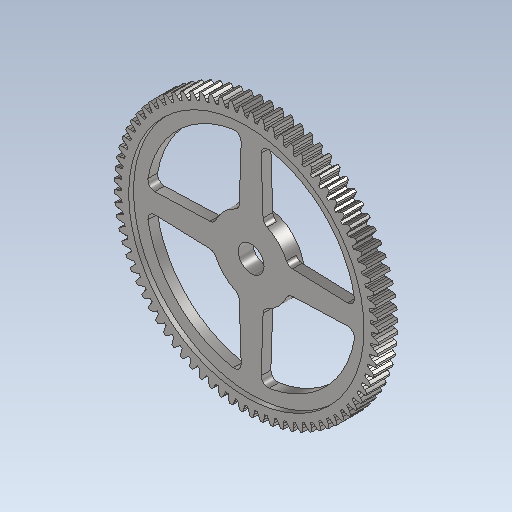
# Autodesk Inventor part: ｍ0.5歯数80焼結ギアd4
Saved by Autodesk Inventor 2020.2 (Build 242310000, 310)
## iProperties
Created: 2020-02-25
Part Number: ｍ0.5歯数80焼結ギアd4
Material: 鋼、炭素鋼
Document SubType Name: Modeling
Designer: aoyam
Density: 7.85 g/cm^3
Appearance: 半つや出し
Mass: 10.8522 g
Surface Area: 26.0429 cm^2
Volume: 1.38245 cm^3
Author: aoyam
Autodesk Inventor part; units mm, degrees
(part 1 of 4)
ref_plane "YZ Plane" through (0, 0, 0) normal (1, 0, 0) x (0, 1, 0)
ref_plane "XZ Plane" through (0, 0, 0) normal (0, 1, 0) x (-1, 0, 0)
ref_plane "XY Plane" through (0, 0, 0) normal (0, 0, 1) x (1, 0, 0)
sketch "スケッチ1" plane through (0, 0, 0) normal (0, 0, 1) x (1, 0, 0)
  arc A0 (4.5173, 26.1611) -> (4.4289, 25.8607) centre (9.5285, 24.5237) ccw
  arc A1 (4.6511, 26.5317) -> (4.5173, 26.1611) centre (10.6083, 24.1715) ccw
  arc A2 (4.8445, 26.9777) -> (4.6511, 26.5317) centre (11.7052, 23.7374) ccw
  arc A3 (4.0497, 25.8607) -> (3.9613, 26.1611) centre (-1.0499, 24.5237) ccw
  arc A4 (3.9613, 26.1611) -> (3.8275, 26.5317) centre (-2.1297, 24.1715) ccw
  arc A5 (3.8275, 26.5317) -> (3.6341, 26.9777) centre (-3.2265, 23.7374) ccw
  arc A6 (4.4289, 25.8607) -> (4.0497, 25.8607) centre (4.2393, 6.4866) ccw
  arc A7 (3.6341, 26.9777) -> (3.2349, 26.962) centre (4.2393, 6.4866) ccw
  arc A8 (2.9728, 26.1223) -> (2.9083, 25.8158) centre (8.097, 24.8831) ccw
  arc A9 (3.0771, 26.5022) -> (2.9728, 26.1223) centre (9.2011, 24.6167) ccw
  arc A10 (3.2349, 26.962) -> (3.0771, 26.5022) centre (10.3287, 24.27) ccw
  arc A11 (2.0283, 26.867) -> (1.6316, 26.8201) centre (4.2393, 6.4866) ccw
  arc A12 (2.2561, 26.4376) -> (2.0283, 26.867) centre (-4.557, 23.0985) ccw
  arc A13 (2.4185, 26.0787) -> (2.2561, 26.4376) centre (-3.4976, 23.6173) ccw
  arc A14 (2.9083, 25.8158) -> (2.5302, 25.7861) centre (4.2393, 6.4866) ccw
  arc A15 (2.5302, 25.7861) -> (2.4185, 26.0787) centre (-2.4488, 24.0531) ccw
  arc A16 (1.4361, 25.9624) -> (1.3958, 25.6518) centre (6.6418, 25.1291) ccw
  arc A17 (1.5103, 26.3493) -> (1.4361, 25.9624) centre (7.7634, 24.9501) ccw
  arc A18 (1.6316, 26.8201) -> (1.5103, 26.3493) centre (8.9146, 24.693) ccw
  arc A19 (0.436, 26.6307) -> (0.0443, 26.5528) centre (4.2393, 6.4866) ccw
  arc A20 (0.6968, 26.2205) -> (0.436, 26.6307) centre (-5.8332, 22.3571) ccw
  arc A21 (0.887, 25.8754) -> (0.6968, 26.2205) centre (-4.8178, 22.9575) ccw
  arc A22 (1.3958, 25.6518) -> (1.0212, 25.5925) centre (4.2393, 6.4866) ccw
  arc A23 (1.0212, 25.5925) -> (0.887, 25.8754) centre (-3.8064, 23.4742) ccw
  arc A24 (-0.0833, 25.6824) -> (-0.0991, 25.3697) centre (5.1717, 25.2601) ccw
  arc A25 (-0.0397, 26.074) -> (-0.0833, 25.6824) centre (6.3039, 25.1697) ccw
  arc A26 (0.0443, 26.5528) -> (-0.0397, 26.074) centre (7.4718, 25.0037) ccw
  arc A27 (-1.1327, 26.2702) -> (-1.5172, 26.1618) centre (4.2393, 6.4866) ccw
  arc A28 (-0.8405, 25.8817) -> (-1.1327, 26.2702) centre (-7.0474, 21.5179) ccw
  arc A29 (-0.6239, 25.5526) -> (-0.8405, 25.8817) centre (-6.0822, 22.1961) ccw
  arc A30 (-0.0991, 25.3697) -> (-0.4679, 25.2811) centre (4.2393, 6.4866) ccw
  arc A31 (-0.4679, 25.2811) -> (-0.6239, 25.5526) centre (-5.1144, 22.7906) ccw
  arc A32 (-1.576, 25.2841) -> (-1.5673, 24.9711) centre (3.6959, 25.2754) ccw
  arc A33 (-1.5633, 25.6779) -> (-1.576, 25.2841) centre (4.8317, 25.2741) ccw
  arc A34 (-1.5172, 26.1618) -> (-1.5633, 25.6779) centre (6.009, 25.2002) ccw
  arc A35 (-2.6684, 25.7878) -> (-3.0431, 25.6495) centre (4.2393, 6.4866) ccw
  arc A36 (-2.3466, 25.4234) -> (-2.6684, 25.7878) centre (-8.1919, 20.5861) ccw
  arc A37 (-2.1048, 25.1123) -> (-2.3466, 25.4234) centre (-7.2829, 21.3378) ccw
  arc A38 (-1.5673, 24.9711) -> (-1.928, 24.8539) centre (4.2393, 6.4866) ccw
  arc A39 (-1.928, 24.8539) -> (-2.1048, 25.1123) centre (-6.3648, 22.0065) ccw
  arc A40 (-3.033, 24.7699) -> (-2.9996, 24.4585) centre (2.2234, 25.1748) ccw
  arc A41 (-3.0512, 25.1635) -> (-3.033, 24.7699) centre (3.3558, 25.2627) ccw
  arc A42 (-3.0431, 25.6495) -> (-3.0512, 25.1635) centre (4.5353, 25.2814) ccw
  arc A43 (-4.1614, 25.1863) -> (-4.5242, 25.0191) centre (4.2393, 6.4866) ccw
  arc A44 (-3.8121, 24.8483) -> (-4.1614, 25.1863) centre (-9.2598, 19.5672) ccw
  arc A45 (-3.5466, 24.5571) -> (-3.8121, 24.8483) centre (-8.4126, 20.388) ccw
  arc A46 (-2.9996, 24.4585) -> (-3.35, 24.3134) centre (4.2393, 6.4866) ccw
  arc A47 (-3.35, 24.3134) -> (-3.5466, 24.5571) centre (-7.5498, 21.1266) ccw
  arc A48 (-4.445, 24.143) -> (-4.3874, 23.8351) centre (0.7634, 24.9591) ccw
  arc A49 (-4.4941, 24.5339) -> (-4.445, 24.143) centre (1.8854, 25.1355) ccw
  arc A50 (-4.5242, 25.0191) -> (-4.4941, 24.5339) centre (3.0597, 25.2466) ccw
  arc A51 (-5.6027, 24.4695) -> (-5.9512, 24.2743) centre (4.2393, 6.4866) ccw
  arc A52 (-5.2279, 24.16) -> (-5.6027, 24.4695) centre (-10.2445, 18.4678) ccw
  arc A53 (-4.9404, 23.8905) -> (-5.2279, 24.16) centre (-9.4643, 19.3525) ccw
  arc A54 (-4.3874, 23.8351) -> (-4.7253, 23.663) centre (4.2393, 6.4866) ccw
  arc A55 (-4.7253, 23.663) -> (-4.9404, 23.8905) centre (-8.6621, 20.1566) ccw
  arc A56 (-5.8036, 23.4072) -> (-5.7219, 23.1048) centre (-0.6753, 24.6294) ccw
  arc A57 (-5.8831, 23.793) -> (-5.8036, 23.4072) centre (0.4294, 24.8933) ccw
  arc A58 (-5.9512, 24.2743) -> (-5.8831, 23.793) centre (1.5915, 25.0963) ccw
  arc A59 (-6.9833, 23.6419) -> (-7.3154, 23.42) centre (4.2393, 6.4866) ccw
  arc A60 (-6.5853, 23.3627) -> (-6.9833, 23.6419) centre (-11.1399, 17.2945) ccw
  arc A61 (-6.2776, 23.1166) -> (-6.5853, 23.3627) centre (-10.4315, 18.2377) ccw
  arc A62 (-5.7219, 23.1048) -> (-6.0453, 22.9067) centre (4.2393, 6.4866) ccw
  arc A63 (-6.0453, 22.9067) -> (-6.2776, 23.1166) centre (-9.6948, 19.1022) ccw
  arc A64 (-7.1002, 22.567) -> (-6.9951, 22.272) centre (-2.0836, 24.1879) ccw
  arc A65 (-7.2097, 22.9455) -> (-7.1002, 22.567) centre (-1.003, 24.5376) ccw
  arc A66 (-7.3154, 23.42) -> (-7.2097, 22.9455) centre (0.1395, 24.8311) ccw
  arc A67 (-8.2947, 22.7085) -> (-8.6084, 22.4612) centre (4.2393, 6.4866) ccw
  arc A68 (-7.876, 22.4614) -> (-8.2947, 22.7085) centre (-11.9405, 16.0545) ccw
  arc A69 (-7.55, 22.2402) -> (-7.876, 22.4614) centre (-11.3083, 17.0504) ccw
  arc A70 (-6.9951, 22.272) -> (-7.3019, 22.0491) centre (4.2393, 6.4866) ccw
  arc A71 (-7.3019, 22.0491) -> (-7.55, 22.2402) centre (-10.6417, 17.97) ccw
  arc A72 (-8.3269, 21.6278) -> (-8.199, 21.3419) centre (-3.4529, 23.6372) ccw
  arc A73 (-8.4658, 21.9965) -> (-8.3269, 21.6278) centre (-2.4031, 24.0707) ccw
  arc A74 (-8.6084, 22.4612) -> (-8.4658, 21.9965) centre (-1.2871, 24.4529) ccw
  arc A75 (-9.5288, 21.6751) -> (-9.8221, 21.4039) centre (4.2393, 6.4866) ccw
  arc A76 (-9.0921, 21.4616) -> (-9.5288, 21.6751) centre (-12.6413, 14.7556) ccw
  arc A77 (-8.7497, 21.2667) -> (-9.0921, 21.4616) centre (-12.0892, 15.798) ccw
  arc A78 (-8.199, 21.3419) -> (-8.4873, 21.0956) centre (4.2393, 6.4866) ccw
  arc A79 (-8.4873, 21.0956) -> (-8.7497, 21.2667) centre (-11.4968, 16.7671) ccw
  arc A80 (-9.4761, 20.5952) -> (-9.3261, 20.3202) centre (-4.7748, 22.9808) ccw
  arc A81 (-9.6435, 20.9518) -> (-9.4761, 20.5952) centre (-3.7622, 23.4953) ccw
  arc A82 (-9.8221, 21.4039) -> (-9.6435, 20.9518) centre (-2.6797, 23.964) ccw
  arc A83 (-10.678, 20.548) -> (-10.9492, 20.2547) centre (4.2393, 6.4866) ccw
  arc A84 (-10.2259, 20.3695) -> (-10.678, 20.548) centre (-13.238, 13.4056) ccw
  arc A85 (-9.8693, 20.202) -> (-10.2259, 20.3695) centre (-12.7694, 14.4882) ccw
  arc A86 (-9.3261, 20.3202) -> (-9.5943, 20.0521) centre (4.2393, 6.4866) ccw
  arc A87 (-9.5943, 20.0521) -> (-9.8693, 20.202) centre (-12.2549, 15.5007) ccw
  arc A88 (-10.5408, 19.4756) -> (-10.3697, 19.2133) centre (-6.0411, 22.2227) ccw
  arc A89 (-10.7357, 19.818) -> (-10.5408, 19.4756) centre (-5.0721, 22.8151) ccw
  arc A90 (-10.9492, 20.2547) -> (-10.7357, 19.818) centre (-4.0296, 23.3672) ccw
  arc A91 (-11.7353, 19.3343) -> (-11.9826, 19.0206) centre (4.2393, 6.4866) ccw
  arc A92 (-11.2705, 19.1917) -> (-11.7353, 19.3343) centre (-13.727, 12.0131) ccw
  arc A93 (-10.9019, 19.0528) -> (-11.2705, 19.1917) centre (-13.3447, 13.129) ccw
  arc A94 (-10.3697, 19.2133) -> (-10.616, 18.9249) centre (4.2393, 6.4866) ccw
  arc A95 (-10.616, 18.9249) -> (-10.9019, 19.0528) centre (-12.9113, 14.1788) ccw
  arc A96 (-11.5143, 18.2759) -> (-11.3232, 18.0278) centre (-7.2441, 21.3676) ccw
  arc A97 (-11.7355, 18.602) -> (-11.5143, 18.2759) centre (-6.3245, 22.0342) ccw
  arc A98 (-11.9826, 19.0206) -> (-11.7355, 18.602) centre (-5.3286, 22.6664) ccw
  arc A99 (-12.694, 18.0413) -> (-12.916, 17.7092) centre (4.2393, 6.4866) ccw
  arc A100 (-12.2196, 17.9357) -> (-12.694, 18.0413) centre (-14.1052, 10.5864) ccw
  arc A101 (-11.8411, 17.8261) -> (-12.2196, 17.9357) centre (-13.8117, 11.7289) ccw
  arc A102 (-11.3232, 18.0278) -> (-11.5461, 17.721) centre (4.2393, 6.4866) ccw
  arc A103 (-11.5461, 17.721) -> (-11.8411, 17.8261) centre (-13.4619, 12.8095) ccw
  arc A104 (-12.3907, 17.0036) -> (-12.1807, 16.7712) centre (-8.3762, 20.4208) ccw
  arc A105 (-12.6368, 17.3113) -> (-12.3907, 17.0036) centre (-7.5118, 21.1574) ccw
  arc A106 (-12.916, 17.7092) -> (-12.6368, 17.3113) centre (-6.5685, 21.8658) ccw
  arc A107 (-13.5484, 16.6771) -> (-13.7436, 16.3286) centre (4.2393, 6.4866) ccw
  arc A108 (-13.0671, 16.609) -> (-13.5484, 16.6771) centre (-14.3703, 9.1345) ccw
  arc A109 (-12.6812, 16.5295) -> (-13.0671, 16.609) centre (-14.1674, 10.2965) ccw
  arc A110 (-12.1807, 16.7712) -> (-12.3789, 16.4479) centre (4.2393, 6.4866) ccw
  arc A111 (-12.3789, 16.4479) -> (-12.6812, 16.5295) centre (-13.9035, 11.4012) ccw
  arc A112 (-13.1646, 15.6664) -> (-12.937, 15.4512) centre (-9.4306, 19.388) ccw
  arc A113 (-13.434, 15.9538) -> (-13.1646, 15.6664) centre (-8.6266, 20.1902) ccw
  arc A114 (-13.7436, 16.3286) -> (-13.434, 15.9538) centre (-7.7419, 20.9705) ccw
  arc A115 (-14.2931, 15.2501) -> (-14.4604, 14.8874) centre (4.2393, 6.4866) ccw
  arc A116 (-13.8079, 15.22) -> (-14.2931, 15.2501) centre (-14.5207, 7.6662) ccw
  arc A117 (-13.417, 15.171) -> (-13.8079, 15.22) centre (-14.4095, 8.8406) ccw
  arc A118 (-12.937, 15.4512) -> (-13.1092, 15.1133) centre (4.2393, 6.4866) ccw
  arc A119 (-13.1092, 15.1133) -> (-13.417, 15.171) centre (-14.2331, 9.9626) ccw
  arc A120 (-13.8312, 14.2726) -> (-13.5874, 14.076) centre (-10.4007, 18.2757) ccw
  arc A121 (-14.1223, 14.538) -> (-13.8312, 14.2726) centre (-9.6621, 19.1385) ccw
  arc A122 (-14.4604, 14.8874) -> (-14.1223, 14.538) centre (-8.8413, 19.9858) ccw
  arc A123 (-14.9236, 13.7691) -> (-15.0618, 13.3943) centre (4.2393, 6.4866) ccw
  arc A124 (-14.4375, 13.7771) -> (-14.9236, 13.7691) centre (-14.5554, 6.1907) ccw
  arc A125 (-14.044, 13.7589) -> (-14.4375, 13.7771) centre (-14.5367, 7.3701) ccw
  arc A126 (-13.5874, 14.076) -> (-13.7326, 13.7256) centre (4.2393, 6.4866) ccw
  arc A127 (-13.7326, 13.7256) -> (-14.044, 13.7589) centre (-14.4489, 8.5025) ccw
  arc A128 (-14.3864, 12.8308) -> (-14.1279, 12.6539) centre (-11.2805, 17.0907) ccw
  arc A129 (-14.6974, 13.0725) -> (-14.3864, 12.8308) centre (-10.6119, 18.0089) ccw
  arc A130 (-15.0618, 13.3943) -> (-14.6974, 13.0725) centre (-9.8601, 18.9179) ccw
  arc A131 (-15.4359, 12.2431) -> (-15.5443, 11.8587) centre (4.2393, 6.4866) ccw
  arc A132 (-14.9519, 12.2893) -> (-15.4359, 12.2431) centre (-14.4743, 4.717) ccw
  arc A133 (-14.5582, 12.302) -> (-14.9519, 12.2893) centre (-14.5482, 5.8943) ccw
  arc A134 (-14.1279, 12.6539) -> (-14.2451, 12.2932) centre (4.2393, 6.4866) ccw
  arc A135 (-14.2451, 12.2932) -> (-14.5582, 12.302) centre (-14.5494, 7.0301) ccw
  arc A136 (-14.8267, 11.3499) -> (-14.5552, 11.1938) centre (-12.0647, 15.8404) ccw
  arc A137 (-15.1558, 11.5665) -> (-14.8267, 11.3499) centre (-11.4701, 16.8081) ccw
  arc A138 (-15.5443, 11.8587) -> (-15.1558, 11.5665) centre (-10.792, 17.7733) ccw
  arc A139 (-15.8269, 10.6817) -> (-15.9048, 10.2899) centre (4.2393, 6.4866) ccw
  arc A140 (-15.3481, 10.7656) -> (-15.8269, 10.6817) centre (-14.2777, 3.2542) ccw
  arc A141 (-14.9565, 10.8092) -> (-15.3481, 10.7656) centre (-14.4438, 4.422) ccw
  arc A142 (-14.5552, 11.1938) -> (-14.6437, 10.825) centre (4.2393, 6.4866) ccw
  arc A143 (-14.6437, 10.825) -> (-14.9565, 10.8092) centre (-14.5342, 5.5542) ccw
  arc A144 (-15.1495, 9.839) -> (-14.8666, 9.7047) centre (-12.7483, 14.5323) ccw
  arc A145 (-15.4946, 10.0291) -> (-15.1495, 9.839) centre (-12.2315, 15.5438) ccw
  arc A146 (-15.9048, 10.2899) -> (-15.4946, 10.0291) centre (-11.6312, 16.5592) ccw
  arc A147 (-16.0942, 9.0944) -> (-16.1411, 8.6977) centre (4.2393, 6.4866) ccw
  arc A148 (-15.6234, 9.2156) -> (-16.0942, 9.0944) centre (-13.967, 1.8113) ccw
  arc A149 (-15.2365, 9.2898) -> (-15.6234, 9.2156) centre (-14.2242, 2.9626) ccw
  arc A150 (-14.8666, 9.7047) -> (-14.9259, 9.3301) centre (4.2393, 6.4866) ccw
  arc A151 (-14.9259, 9.3301) -> (-15.2365, 9.2898) centre (-14.4031, 4.0842) ccw
  arc A152 (-15.3527, 8.3074) -> (-15.0602, 8.1957) centre (-13.3272, 13.1747) ccw
  arc A153 (-15.7117, 8.4699) -> (-15.3527, 8.3074) centre (-12.8914, 14.2235) ccw
  arc A154 (-16.1411, 8.6977) -> (-15.7117, 8.4699) centre (-12.3726, 15.2829) ccw
  arc A155 (-16.2361, 7.491) -> (-16.2518, 7.0918) centre (4.2393, 6.4866) ccw
  arc A156 (-15.7763, 7.6488) -> (-16.2361, 7.491) centre (-13.5441, 0.3973) ccw
  arc A157 (-15.3964, 7.7531) -> (-15.7763, 7.6488) centre (-13.8908, 1.5248) ccw
  arc A158 (-15.0602, 8.1957) -> (-15.0899, 7.8177) centre (4.2393, 6.4866) ccw
  arc A159 (-15.0899, 7.8177) -> (-15.3964, 7.7531) centre (-14.1572, 2.6289) ccw
  arc A160 (-15.4352, 6.7646) -> (-15.1348, 6.6762) centre (-13.7978, 11.7758) ccw
  arc A161 (-15.8058, 6.8984) -> (-15.4352, 6.7646) centre (-13.4456, 12.8556) ccw
  arc A162 (-16.2518, 7.0918) -> (-15.8058, 6.8984) centre (-13.0115, 13.9525) ccw
  arc A163 (-16.2518, 5.8814) -> (-16.2361, 5.4823) centre (4.2393, 6.4866) ccw
  arc A164 (-15.8058, 6.0748) -> (-16.2518, 5.8814) centre (-13.0115, -0.9792) ccw
  arc A165 (-15.4352, 6.2086) -> (-15.8058, 6.0748) centre (-13.4456, 0.1176) ccw
  arc A166 (-15.1348, 6.6762) -> (-15.1348, 6.297) centre (4.2393, 6.4866) ccw
  arc A167 (-15.1348, 6.297) -> (-15.4352, 6.2086) centre (-13.7978, 1.1974) ccw
  arc A168 (-15.3964, 5.2201) -> (-15.0899, 5.1556) centre (-14.1572, 10.3443) ccw
  arc A169 (-15.7763, 5.3244) -> (-15.3964, 5.2201) centre (-13.8908, 11.4485) ccw
  arc A170 (-16.2361, 5.4823) -> (-15.7763, 5.3244) centre (-13.5441, 12.576) ccw
  arc A171 (-16.1411, 4.2756) -> (-16.0942, 3.8789) centre (4.2393, 6.4866) ccw
  arc A172 (-15.7117, 4.5034) -> (-16.1411, 4.2756) centre (-12.3726, -2.3097) ccw
  arc A173 (-15.3527, 4.6658) -> (-15.7117, 4.5034) centre (-12.8914, -1.2503) ccw
  arc A174 (-15.0899, 5.1556) -> (-15.0602, 4.7775) centre (4.2393, 6.4866) ccw
  arc A175 (-15.0602, 4.7775) -> (-15.3527, 4.6658) centre (-13.3272, -0.2015) ccw
  arc A176 (-15.2365, 3.6834) -> (-14.9259, 3.6431) centre (-14.4031, 8.8891) ccw
  arc A177 (-15.6234, 3.7576) -> (-15.2365, 3.6834) centre (-14.2242, 10.0107) ccw
  arc A178 (-16.0942, 3.8789) -> (-15.6234, 3.7576) centre (-13.967, 11.1619) ccw
  arc A179 (-15.9048, 2.6834) -> (-15.8269, 2.2916) centre (4.2393, 6.4866) ccw
  arc A180 (-15.4946, 2.9442) -> (-15.9048, 2.6834) centre (-11.6312, -3.5859) ccw
  arc A181 (-15.1495, 3.1343) -> (-15.4946, 2.9442) centre (-12.2315, -2.5705) ccw
  arc A182 (-14.9259, 3.6431) -> (-14.8666, 3.2686) centre (4.2393, 6.4866) ccw
  arc A183 (-14.8666, 3.2686) -> (-15.1495, 3.1343) centre (-12.7483, -1.5591) ccw
  arc A184 (-14.9565, 2.164) -> (-14.6437, 2.1482) centre (-14.5342, 7.419) ccw
  arc A185 (-15.3481, 2.2076) -> (-14.9565, 2.164) centre (-14.4438, 8.5512) ccw
  arc A186 (-15.8269, 2.2916) -> (-15.3481, 2.2076) centre (-14.2777, 9.7191) ccw
  arc A187 (-15.5443, 1.1146) -> (-15.4359, 0.7301) centre (4.2393, 6.4866) ccw
  arc A188 (-15.1558, 1.4068) -> (-15.5443, 1.1146) centre (-10.792, -4.8001) ccw
  arc A189 (-14.8267, 1.6234) -> (-15.1558, 1.4068) centre (-11.4701, -3.8349) ccw
  arc A190 (-14.6437, 2.1482) -> (-14.5552, 1.7794) centre (4.2393, 6.4866) ccw
  arc A191 (-14.5552, 1.7794) -> (-14.8267, 1.6234) centre (-12.0647, -2.8671) ccw
  arc A192 (-14.5582, 0.6713) -> (-14.2451, 0.6801) centre (-14.5494, 5.9432) ccw
  arc A193 (-14.9519, 0.684) -> (-14.5582, 0.6713) centre (-14.5482, 7.079) ccw
  arc A194 (-15.4359, 0.7301) -> (-14.9519, 0.684) centre (-14.4743, 8.2563) ccw
  arc A195 (-15.0618, -0.4211) -> (-14.9236, -0.7958) centre (4.2393, 6.4866) ccw
  arc A196 (-14.6974, -0.0993) -> (-15.0618, -0.4211) centre (-9.8601, -5.9446) ccw
  arc A197 (-14.3864, 0.1425) -> (-14.6974, -0.0993) centre (-10.6119, -5.0356) ccw
  arc A198 (-14.2451, 0.6801) -> (-14.1279, 0.3194) centre (4.2393, 6.4866) ccw
  arc A199 (-14.1279, 0.3194) -> (-14.3864, 0.1425) centre (-11.2805, -4.1175) ccw
  arc A200 (-14.044, -0.7856) -> (-13.7326, -0.7523) centre (-14.4489, 4.4707) ccw
  arc A201 (-14.4375, -0.8038) -> (-14.044, -0.7856) centre (-14.5367, 5.6031) ccw
  arc A202 (-14.9236, -0.7958) -> (-14.4375, -0.8038) centre (-14.5554, 6.7826) ccw
  arc A203 (-14.4604, -1.9141) -> (-14.2931, -2.2769) centre (4.2393, 6.4866) ccw
  arc A204 (-14.1223, -1.5647) -> (-14.4604, -1.9141) centre (-8.8413, -7.0125) ccw
  arc A205 (-13.8312, -1.2993) -> (-14.1223, -1.5647) centre (-9.6621, -6.1653) ccw
  arc A206 (-13.7326, -0.7523) -> (-13.5874, -1.1027) centre (4.2393, 6.4866) ccw
  arc A207 (-13.5874, -1.1027) -> (-13.8312, -1.2993) centre (-10.4007, -5.3025) ccw
  arc A208 (-13.417, -2.1977) -> (-13.1092, -2.1401) centre (-14.2331, 3.0107) ccw
  arc A209 (-13.8079, -2.2467) -> (-13.417, -2.1977) centre (-14.4095, 4.1327) ccw
  arc A210 (-14.2931, -2.2769) -> (-13.8079, -2.2467) centre (-14.5207, 5.307) ccw
  arc A211 (-13.7436, -3.3554) -> (-13.5484, -3.7039) centre (4.2393, 6.4866) ccw
  arc A212 (-13.434, -2.9806) -> (-13.7436, -3.3554) centre (-7.7419, -7.9972) ccw
  arc A213 (-13.1646, -2.6931) -> (-13.434, -2.9806) centre (-8.6266, -7.217) ccw
  arc A214 (-13.1092, -2.1401) -> (-12.937, -2.478) centre (4.2393, 6.4866) ccw
  arc A215 (-12.937, -2.478) -> (-13.1646, -2.6931) centre (-9.4306, -6.4148) ccw
  arc A216 (-12.6812, -3.5562) -> (-12.3789, -3.4746) centre (-13.9035, 1.5721) ccw
  arc A217 (-13.0671, -3.6358) -> (-12.6812, -3.5562) centre (-14.1674, 2.6768) ccw
  arc A218 (-13.5484, -3.7039) -> (-13.0671, -3.6358) centre (-14.3703, 3.8388) ccw
  arc A219 (-12.916, -4.736) -> (-12.694, -5.0681) centre (4.2393, 6.4866) ccw
  arc A220 (-12.6368, -4.338) -> (-12.916, -4.736) centre (-6.5685, -8.8926) ccw
  arc A221 (-12.3907, -4.0303) -> (-12.6368, -4.338) centre (-7.5118, -8.1842) ccw
  arc A222 (-12.3789, -3.4746) -> (-12.1807, -3.798) centre (4.2393, 6.4866) ccw
  arc A223 (-12.1807, -3.798) -> (-12.3907, -4.0303) centre (-8.3762, -7.4475) ccw
  arc A224 (-11.8411, -4.8528) -> (-11.5461, -4.7478) centre (-13.4619, 0.1637) ccw
  arc A225 (-12.2196, -4.9624) -> (-11.8411, -4.8528) centre (-13.8117, 1.2443) ccw
  arc A226 (-12.694, -5.0681) -> (-12.2196, -4.9624) centre (-14.1052, 2.3868) ccw
  arc A227 (-11.9826, -6.0473) -> (-11.7353, -6.3611) centre (4.2393, 6.4866) ccw
  arc A228 (-11.7355, -5.6287) -> (-11.9826, -6.0473) centre (-5.3286, -9.6932) ccw
  arc A229 (-11.5143, -5.3027) -> (-11.7355, -5.6287) centre (-6.3245, -9.0609) ccw
  arc A230 (-11.5461, -4.7478) -> (-11.3232, -5.0546) centre (4.2393, 6.4866) ccw
  arc A231 (-11.3232, -5.0546) -> (-11.5143, -5.3027) centre (-7.2441, -8.3944) ccw
  arc A232 (-10.9019, -6.0795) -> (-10.616, -5.9516) centre (-12.9113, -1.2056) ccw
  arc A233 (-11.2705, -6.2185) -> (-10.9019, -6.0795) centre (-13.3447, -0.1558) ccw
  arc A234 (-11.7353, -6.3611) -> (-11.2705, -6.2185) centre (-13.727, 0.9602) ccw
  arc A235 (-10.9492, -7.2815) -> (-10.678, -7.5748) centre (4.2393, 6.4866) ccw
  arc A236 (-10.7357, -6.8447) -> (-10.9492, -7.2815) centre (-4.0296, -10.394) ccw
  arc A237 (-10.5408, -6.5023) -> (-10.7357, -6.8447) centre (-5.0721, -9.8418) ccw
  arc A238 (-10.616, -5.9516) -> (-10.3697, -6.24) centre (4.2393, 6.4866) ccw
  arc A239 (-10.3697, -6.24) -> (-10.5408, -6.5023) centre (-6.0411, -9.2495) ccw
  arc A240 (-9.8693, -7.2288) -> (-9.5943, -7.0788) centre (-12.2549, -2.5275) ccw
  arc A241 (-10.2259, -7.3962) -> (-9.8693, -7.2288) centre (-12.7694, -1.5149) ccw
  arc A242 (-10.678, -7.5748) -> (-10.2259, -7.3962) centre (-13.238, -0.4324) ccw
  arc A243 (-9.8221, -8.4307) -> (-9.5288, -8.7019) centre (4.2393, 6.4866) ccw
  arc A244 (-9.6435, -7.9786) -> (-9.8221, -8.4307) centre (-2.6797, -10.9907) ccw
  arc A245 (-9.4761, -7.6219) -> (-9.6435, -7.9786) centre (-3.7622, -10.5221) ccw
  arc A246 (-9.5943, -7.0788) -> (-9.3261, -7.347) centre (4.2393, 6.4866) ccw
  arc A247 (-9.3261, -7.347) -> (-9.4761, -7.6219) centre (-4.7748, -10.0076) ccw
  arc A248 (-8.7497, -8.2934) -> (-8.4873, -8.1224) centre (-11.4968, -3.7938) ccw
  arc A249 (-9.0921, -8.4883) -> (-8.7497, -8.2934) centre (-12.0892, -2.8247) ccw
  arc A250 (-9.5288, -8.7019) -> (-9.0921, -8.4883) centre (-12.6413, -1.7823) ccw
  arc A251 (-8.6084, -9.488) -> (-8.2947, -9.7353) centre (4.2393, 6.4866) ccw
  arc A252 (-8.4658, -9.0232) -> (-8.6084, -9.488) centre (-1.2871, -11.4797) ccw
  arc A253 (-8.3269, -8.6545) -> (-8.4658, -9.0232) centre (-2.4031, -11.0974) ccw
  arc A254 (-8.4873, -8.1224) -> (-8.199, -8.3687) centre (4.2393, 6.4866) ccw
  arc A255 (-8.199, -8.3687) -> (-8.3269, -8.6545) centre (-3.4529, -10.664) ccw
  arc A256 (-7.55, -9.267) -> (-7.3019, -9.0759) centre (-10.6417, -4.9968) ccw
  arc A257 (-7.876, -9.4881) -> (-7.55, -9.267) centre (-11.3083, -4.0772) ccw
  arc A258 (-8.2947, -9.7353) -> (-7.876, -9.4881) centre (-11.9405, -3.0813) ccw
  arc A259 (-7.3154, -10.4467) -> (-6.9833, -10.6687) centre (4.2393, 6.4866) ccw
  arc A260 (-7.2097, -9.9722) -> (-7.3154, -10.4467) centre (0.1395, -11.8579) ccw
  arc A261 (-7.1002, -9.5938) -> (-7.2097, -9.9722) centre (-1.003, -11.5644) ccw
  arc A262 (-7.3019, -9.0759) -> (-6.9951, -9.2988) centre (4.2393, 6.4866) ccw
  arc A263 (-6.9951, -9.2988) -> (-7.1002, -9.5938) centre (-2.0836, -11.2146) ccw
  arc A264 (-6.2776, -10.1434) -> (-6.0453, -9.9334) centre (-9.6948, -6.1289) ccw
  arc A265 (-6.5853, -10.3895) -> (-6.2776, -10.1434) centre (-10.4315, -5.2644) ccw
  arc A266 (-6.9833, -10.6687) -> (-6.5853, -10.3895) centre (-11.1399, -4.3212) ccw
  arc A267 (-5.9512, -11.3011) -> (-5.6027, -11.4963) centre (4.2393, 6.4866) ccw
  arc A268 (-5.8831, -10.8198) -> (-5.9512, -11.3011) centre (1.5915, -12.123) ccw
  arc A269 (-5.8036, -10.4339) -> (-5.8831, -10.8198) centre (0.4294, -11.92) ccw
  arc A270 (-6.0453, -9.9334) -> (-5.7219, -10.1316) centre (4.2393, 6.4866) ccw
  arc A271 (-5.7219, -10.1316) -> (-5.8036, -10.4339) centre (-0.6753, -11.6561) ccw
  arc A272 (-4.9404, -10.9173) -> (-4.7253, -10.6897) centre (-8.6621, -7.1833) ccw
  arc A273 (-5.2279, -11.1867) -> (-4.9404, -10.9173) centre (-9.4643, -6.3793) ccw
  arc A274 (-5.6027, -11.4963) -> (-5.2279, -11.1867) centre (-10.2445, -5.4945) ccw
  arc A275 (-4.5242, -12.0458) -> (-4.1614, -12.213) centre (4.2393, 6.4866) ccw
  arc A276 (-4.4941, -11.5606) -> (-4.5242, -12.0458) centre (3.0597, -12.2734) ccw
  arc A277 (-4.445, -11.1697) -> (-4.4941, -11.5606) centre (1.8854, -12.1622) ccw
  arc A278 (-4.7253, -10.6897) -> (-4.3874, -10.8619) centre (4.2393, 6.4866) ccw
  arc A279 (-4.3874, -10.8619) -> (-4.445, -11.1697) centre (0.7634, -11.9858) ccw
  arc A280 (-3.5466, -11.5839) -> (-3.35, -11.3401) centre (-7.5498, -8.1534) ccw
  arc A281 (-3.8121, -11.875) -> (-3.5466, -11.5839) centre (-8.4126, -7.4148) ccw
  arc A282 (-4.1614, -12.213) -> (-3.8121, -11.875) centre (-9.2598, -6.594) ccw
  arc A283 (-3.0431, -12.6763) -> (-2.6684, -12.8145) centre (4.2393, 6.4866) ccw
  arc A284 (-3.0512, -12.1902) -> (-3.0431, -12.6763) centre (4.5353, -12.3081) ccw
  arc A285 (-3.033, -11.7966) -> (-3.0512, -12.1902) centre (3.3558, -12.2894) ccw
  arc A286 (-3.35, -11.3401) -> (-2.9996, -11.4853) centre (4.2393, 6.4866) ccw
  arc A287 (-2.9996, -11.4853) -> (-3.033, -11.7966) centre (2.2234, -12.2016) ccw
  arc A288 (-2.1048, -12.139) -> (-1.928, -11.8806) centre (-6.3648, -9.0332) ccw
  arc A289 (-2.3466, -12.4501) -> (-2.1048, -12.139) centre (-7.2829, -8.3646) ccw
  arc A290 (-2.6684, -12.8145) -> (-2.3466, -12.4501) centre (-8.1919, -7.6128) ccw
  arc A291 (-1.5172, -13.1886) -> (-1.1327, -13.297) centre (4.2393, 6.4866) ccw
  arc A292 (-1.5633, -12.7046) -> (-1.5172, -13.1886) centre (6.009, -12.227) ccw
  arc A293 (-1.576, -12.3109) -> (-1.5633, -12.7046) centre (4.8317, -12.3009) ccw
  arc A294 (-1.928, -11.8806) -> (-1.5673, -11.9978) centre (4.2393, 6.4866) ccw
  arc A295 (-1.5673, -11.9978) -> (-1.576, -12.3109) centre (3.6959, -12.3021) ccw
  arc A296 (-0.6239, -12.5794) -> (-0.4679, -12.3079) centre (-5.1144, -9.8174) ccw
  arc A297 (-0.8405, -12.9085) -> (-0.6239, -12.5794) centre (-6.0822, -9.2228) ccw
  arc A298 (-1.1327, -13.297) -> (-0.8405, -12.9085) centre (-7.0474, -8.5447) ccw
  arc A299 (0.0443, -13.5796) -> (0.436, -13.6575) centre (4.2393, 6.4866) ccw
  arc A300 (-0.0397, -13.1007) -> (0.0443, -13.5796) centre (7.4718, -12.0304) ccw
  arc A301 (-0.0833, -12.7092) -> (-0.0397, -13.1007) centre (6.3039, -12.1965) ccw
  arc A302 (-0.4679, -12.3079) -> (-0.0991, -12.3964) centre (4.2393, 6.4866) ccw
  arc A303 (-0.0991, -12.3964) -> (-0.0833, -12.7092) centre (5.1717, -12.2869) ccw
  arc A304 (0.887, -12.9022) -> (1.0212, -12.6193) centre (-3.8064, -10.501) ccw
  arc A305 (0.6968, -13.2473) -> (0.887, -12.9022) centre (-4.8178, -9.9842) ccw
  arc A306 (0.436, -13.6575) -> (0.6968, -13.2473) centre (-5.8332, -9.3839) ccw
  arc A307 (1.6316, -13.8468) -> (2.0283, -13.8938) centre (4.2393, 6.4866) ccw
  arc A308 (1.5103, -13.3761) -> (1.6316, -13.8468) centre (8.9146, -11.7197) ccw
  arc A309 (1.4361, -12.9891) -> (1.5103, -13.3761) centre (7.7634, -11.9769) ccw
  arc A310 (1.0212, -12.6193) -> (1.3958, -12.6786) centre (4.2393, 6.4866) ccw
  arc A311 (1.3958, -12.6786) -> (1.4361, -12.9891) centre (6.6418, -12.1558) ccw
  arc A312 (2.4185, -13.1054) -> (2.5302, -12.8128) centre (-2.4488, -11.0799) ccw
  arc A313 (2.2561, -13.4644) -> (2.4185, -13.1054) centre (-3.4976, -10.6441) ccw
  arc A314 (2.0283, -13.8938) -> (2.2561, -13.4644) centre (-4.557, -10.1253) ccw
  arc A315 (3.2349, -13.9888) -> (3.6341, -14.0044) centre (4.2393, 6.4866) ccw
  arc A316 (3.0771, -13.529) -> (3.2349, -13.9888) centre (10.3287, -11.2968) ccw
  arc A317 (2.9728, -13.149) -> (3.0771, -13.529) centre (9.2011, -11.6435) ccw
  arc A318 (2.5302, -12.8128) -> (2.9083, -12.8426) centre (4.2393, 6.4866) ccw
  arc A319 (2.9083, -12.8426) -> (2.9728, -13.149) centre (8.097, -11.9099) ccw
  arc A320 (3.9613, -13.1879) -> (4.0497, -12.8874) centre (-1.0499, -11.5505) ccw
  arc A321 (3.8275, -13.5585) -> (3.9613, -13.1879) centre (-2.1297, -11.1983) ccw
  arc A322 (3.6341, -14.0044) -> (3.8275, -13.5585) centre (-3.2265, -10.7642) ccw
  arc A323 (4.8445, -14.0044) -> (5.2437, -13.9888) centre (4.2393, 6.4866) ccw
  arc A324 (4.6511, -13.5585) -> (4.8445, -14.0044) centre (11.7052, -10.7642) ccw
  arc A325 (4.5173, -13.1879) -> (4.6511, -13.5585) centre (10.6083, -11.1983) ccw
  arc A326 (4.0497, -12.8874) -> (4.4289, -12.8874) centre (4.2393, 6.4866) ccw
  arc A327 (4.4289, -12.8874) -> (4.5173, -13.1879) centre (9.5285, -11.5505) ccw
  arc A328 (5.5058, -13.149) -> (5.5703, -12.8426) centre (0.3816, -11.9099) ccw
  arc A329 (5.4015, -13.529) -> (5.5058, -13.149) centre (-0.7225, -11.6435) ccw
  arc A330 (5.2437, -13.9888) -> (5.4015, -13.529) centre (-1.85, -11.2968) ccw
  arc A331 (6.4504, -13.8938) -> (6.8471, -13.8468) centre (4.2393, 6.4866) ccw
  arc A332 (6.2226, -13.4644) -> (6.4504, -13.8938) centre (13.0356, -10.1253) ccw
  arc A333 (6.0601, -13.1054) -> (6.2226, -13.4644) centre (11.9762, -10.6441) ccw
  arc A334 (5.5703, -12.8426) -> (5.9484, -12.8128) centre (4.2393, 6.4866) ccw
  arc A335 (5.9484, -12.8128) -> (6.0601, -13.1054) centre (10.9274, -11.0799) ccw
  arc A336 (7.0425, -12.9891) -> (7.0828, -12.6786) centre (1.8368, -12.1558) ccw
  arc A337 (6.9683, -13.3761) -> (7.0425, -12.9891) centre (0.7152, -11.9769) ccw
  arc A338 (6.8471, -13.8468) -> (6.9683, -13.3761) centre (-0.436, -11.7197) ccw
  arc A339 (8.0426, -13.6575) -> (8.4344, -13.5796) centre (4.2393, 6.4866) ccw
  arc A340 (7.7818, -13.2473) -> (8.0426, -13.6575) centre (14.3119, -9.3839) ccw
  arc A341 (7.5917, -12.9022) -> (7.7818, -13.2473) centre (13.2964, -9.9842) ccw
  arc A342 (7.0828, -12.6786) -> (7.4574, -12.6193) centre (4.2393, 6.4866) ccw
  arc A343 (7.4574, -12.6193) -> (7.5917, -12.9022) centre (12.285, -10.501) ccw
  arc A344 (8.5619, -12.7092) -> (8.5777, -12.3964) centre (3.3069, -12.2869) ccw
  arc A345 (8.5183, -13.1007) -> (8.5619, -12.7092) centre (2.1747, -12.1965) ccw
  arc A346 (8.4344, -13.5796) -> (8.5183, -13.1007) centre (1.0069, -12.0304) ccw
  arc A347 (9.6113, -13.297) -> (9.9958, -13.1886) centre (4.2393, 6.4866) ccw
  arc A348 (9.3192, -12.9085) -> (9.6113, -13.297) centre (15.526, -8.5447) ccw
  arc A349 (9.1026, -12.5794) -> (9.3192, -12.9085) centre (14.5608, -9.2228) ccw
  arc A350 (8.5777, -12.3964) -> (8.9465, -12.3079) centre (4.2393, 6.4866) ccw
  arc A351 (8.9465, -12.3079) -> (9.1026, -12.5794) centre (13.5931, -9.8174) ccw
  arc A352 (10.0547, -12.3109) -> (10.0459, -11.9978) centre (4.7827, -12.3021) ccw
  arc A353 (10.0419, -12.7046) -> (10.0547, -12.3109) centre (3.647, -12.3009) ccw
  arc A354 (9.9958, -13.1886) -> (10.0419, -12.7046) centre (2.4697, -12.227) ccw
  arc A355 (11.147, -12.8145) -> (11.5218, -12.6763) centre (4.2393, 6.4866) ccw
  arc A356 (10.8252, -12.4501) -> (11.147, -12.8145) centre (16.6706, -7.6128) ccw
  arc A357 (10.5835, -12.139) -> (10.8252, -12.4501) centre (15.7615, -8.3646) ccw
  arc A358 (10.0459, -11.9978) -> (10.4066, -11.8806) centre (4.2393, 6.4866) ccw
  arc A359 (10.4066, -11.8806) -> (10.5835, -12.139) centre (14.8434, -9.0332) ccw
  arc A360 (11.5116, -11.7966) -> (11.4783, -11.4853) centre (6.2552, -12.2016) ccw
  arc A361 (11.5298, -12.1902) -> (11.5116, -11.7966) centre (5.1228, -12.2894) ccw
  arc A362 (11.5218, -12.6763) -> (11.5298, -12.1902) centre (3.9434, -12.3081) ccw
  arc A363 (12.64, -12.213) -> (13.0028, -12.0458) centre (4.2393, 6.4866) ccw
  arc A364 (12.2907, -11.875) -> (12.64, -12.213) centre (17.7385, -6.594) ccw
  arc A365 (12.0253, -11.5839) -> (12.2907, -11.875) centre (16.8912, -7.4148) ccw
  arc A366 (11.4783, -11.4853) -> (11.8286, -11.3401) centre (4.2393, 6.4866) ccw
  arc A367 (11.8286, -11.3401) -> (12.0253, -11.5839) centre (16.0284, -8.1534) ccw
  arc A368 (12.9236, -11.1697) -> (12.866, -10.8619) centre (7.7153, -11.9858) ccw
  arc A369 (12.9727, -11.5606) -> (12.9236, -11.1697) centre (6.5933, -12.1622) ccw
  arc A370 (13.0028, -12.0458) -> (12.9727, -11.5606) centre (5.4189, -12.2734) ccw
  arc A371 (14.0813, -11.4963) -> (14.4298, -11.3011) centre (4.2393, 6.4866) ccw
  arc A372 (13.7065, -11.1867) -> (14.0813, -11.4963) centre (18.7231, -5.4945) ccw
  arc A373 (13.4191, -10.9173) -> (13.7065, -11.1867) centre (17.9429, -6.3793) ccw
  arc A374 (12.866, -10.8619) -> (13.2039, -10.6897) centre (4.2393, 6.4866) ccw
  arc A375 (13.2039, -10.6897) -> (13.4191, -10.9173) centre (17.1407, -7.1833) ccw
  arc A376 (14.2822, -10.4339) -> (14.2006, -10.1316) centre (9.1539, -11.6561) ccw
  arc A377 (14.3617, -10.8198) -> (14.2822, -10.4339) centre (8.0492, -11.92) ccw
  arc A378 (14.4298, -11.3011) -> (14.3617, -10.8198) centre (6.8872, -12.123) ccw
  arc A379 (15.4619, -10.6687) -> (15.794, -10.4467) centre (4.2393, 6.4866) ccw
  arc A380 (15.064, -10.3895) -> (15.4619, -10.6687) centre (19.6185, -4.3212) ccw
  arc A381 (14.7563, -10.1434) -> (15.064, -10.3895) centre (18.9101, -5.2644) ccw
  arc A382 (14.2006, -10.1316) -> (14.5239, -9.9334) centre (4.2393, 6.4866) ccw
  arc A383 (14.5239, -9.9334) -> (14.7563, -10.1434) centre (18.1735, -6.1289) ccw
  arc A384 (15.5788, -9.5938) -> (15.4737, -9.2988) centre (10.5622, -11.2146) ccw
  arc A385 (15.6884, -9.9722) -> (15.5788, -9.5938) centre (9.4816, -11.5644) ccw
  arc A386 (15.794, -10.4467) -> (15.6884, -9.9722) centre (8.3391, -11.8579) ccw
  arc A387 (16.7733, -9.7353) -> (17.087, -9.488) centre (4.2393, 6.4866) ccw
  arc A388 (16.3547, -9.4881) -> (16.7733, -9.7353) centre (20.4191, -3.0813) ccw
  arc A389 (16.0286, -9.267) -> (16.3547, -9.4881) centre (19.7869, -4.0772) ccw
  arc A390 (15.4737, -9.2988) -> (15.7805, -9.0759) centre (4.2393, 6.4866) ccw
  arc A391 (15.7805, -9.0759) -> (16.0286, -9.267) centre (19.1203, -4.9968) ccw
  arc A392 (16.8055, -8.6545) -> (16.6776, -8.3687) centre (11.9315, -10.664) ccw
  arc A393 (16.9444, -9.0232) -> (16.8055, -8.6545) centre (10.8817, -11.0974) ccw
  arc A394 (17.087, -9.488) -> (16.9444, -9.0232) centre (9.7657, -11.4797) ccw
  arc A395 (18.0074, -8.7019) -> (18.3007, -8.4307) centre (4.2393, 6.4866) ccw
  arc A396 (17.5707, -8.4883) -> (18.0074, -8.7019) centre (21.1199, -1.7823) ccw
  arc A397 (17.2283, -8.2934) -> (17.5707, -8.4883) centre (20.5678, -2.8247) ccw
  arc A398 (16.6776, -8.3687) -> (16.966, -8.1224) centre (4.2393, 6.4866) ccw
  arc A399 (16.966, -8.1224) -> (17.2283, -8.2934) centre (19.9754, -3.7938) ccw
  arc A400 (17.9547, -7.6219) -> (17.8048, -7.347) centre (13.2534, -10.0076) ccw
  arc A401 (18.1221, -7.9786) -> (17.9547, -7.6219) centre (12.2409, -10.5221) ccw
  arc A402 (18.3007, -8.4307) -> (18.1221, -7.9786) centre (11.1583, -10.9907) ccw
  arc A403 (19.1566, -7.5748) -> (19.4278, -7.2815) centre (4.2393, 6.4866) ccw
  arc A404 (18.7045, -7.3962) -> (19.1566, -7.5748) centre (21.7166, -0.4324) ccw
  arc A405 (18.3479, -7.2288) -> (18.7045, -7.3962) centre (21.248, -1.5149) ccw
  arc A406 (17.8048, -7.347) -> (18.0729, -7.0788) centre (4.2393, 6.4866) ccw
  arc A407 (18.0729, -7.0788) -> (18.3479, -7.2288) centre (20.7335, -2.5275) ccw
  arc A408 (19.0194, -6.5023) -> (18.8483, -6.24) centre (14.5198, -9.2495) ccw
  arc A409 (19.2143, -6.8447) -> (19.0194, -6.5023) centre (13.5507, -9.8418) ccw
  arc A410 (19.4278, -7.2815) -> (19.2143, -6.8447) centre (12.5083, -10.394) ccw
  arc A411 (20.2139, -6.3611) -> (20.4612, -6.0473) centre (4.2393, 6.4866) ccw
  arc A412 (19.7492, -6.2185) -> (20.2139, -6.3611) centre (22.2056, 0.9602) ccw
  arc A413 (19.3805, -6.0795) -> (19.7492, -6.2185) centre (21.8234, -0.1558) ccw
  arc A414 (18.8483, -6.24) -> (19.0946, -5.9516) centre (4.2393, 6.4866) ccw
  arc A415 (19.0946, -5.9516) -> (19.3805, -6.0795) centre (21.3899, -1.2056) ccw
  arc A416 (19.9929, -5.3027) -> (19.8018, -5.0546) centre (15.7227, -8.3944) ccw
  arc A417 (20.2141, -5.6287) -> (19.9929, -5.3027) centre (14.8031, -9.0609) ccw
  arc A418 (20.4612, -6.0473) -> (20.2141, -5.6287) centre (13.8072, -9.6932) ccw
  arc A419 (21.1727, -5.0681) -> (21.3946, -4.736) centre (4.2393, 6.4866) ccw
  arc A420 (20.6982, -4.9624) -> (21.1727, -5.0681) centre (22.5838, 2.3868) ccw
  arc A421 (20.3197, -4.8528) -> (20.6982, -4.9624) centre (22.2903, 1.2443) ccw
  arc A422 (19.8018, -5.0546) -> (20.0247, -4.7478) centre (4.2393, 6.4866) ccw
  arc A423 (20.0247, -4.7478) -> (20.3197, -4.8528) centre (21.9406, 0.1637) ccw
  arc A424 (20.8693, -4.0303) -> (20.6593, -3.798) centre (16.8549, -7.4475) ccw
  arc A425 (21.1154, -4.338) -> (20.8693, -4.0303) centre (15.9904, -8.1842) ccw
  arc A426 (21.3946, -4.736) -> (21.1154, -4.338) centre (15.0472, -8.8926) ccw
  arc A427 (22.027, -3.7039) -> (22.2222, -3.3554) centre (4.2393, 6.4866) ccw
  arc A428 (21.5457, -3.6358) -> (22.027, -3.7039) centre (22.8489, 3.8388) ccw
  arc A429 (21.1598, -3.5562) -> (21.5457, -3.6358) centre (22.646, 2.6768) ccw
  arc A430 (20.6593, -3.798) -> (20.8575, -3.4746) centre (4.2393, 6.4866) ccw
  arc A431 (20.8575, -3.4746) -> (21.1598, -3.5562) centre (22.3821, 1.5721) ccw
  arc A432 (21.6432, -2.6931) -> (21.4156, -2.478) centre (17.9092, -6.4148) ccw
  arc A433 (21.9127, -2.9806) -> (21.6432, -2.6931) centre (17.1052, -7.217) ccw
  arc A434 (22.2222, -3.3554) -> (21.9127, -2.9806) centre (16.2205, -7.9972) ccw
  arc A435 (22.7717, -2.2769) -> (22.939, -1.9141) centre (4.2393, 6.4866) ccw
  arc A436 (22.2866, -2.2467) -> (22.7717, -2.2769) centre (22.9993, 5.307) ccw
  arc A437 (21.8956, -2.1977) -> (22.2866, -2.2467) centre (22.8881, 4.1327) ccw
  arc A438 (21.4156, -2.478) -> (21.5878, -2.1401) centre (4.2393, 6.4866) ccw
  arc A439 (21.5878, -2.1401) -> (21.8956, -2.1977) centre (22.7117, 3.0107) ccw
  arc A440 (22.3098, -1.2993) -> (22.0661, -1.1027) centre (18.8793, -5.3025) ccw
  arc A441 (22.601, -1.5647) -> (22.3098, -1.2993) centre (18.1407, -6.1653) ccw
  arc A442 (22.939, -1.9141) -> (22.601, -1.5647) centre (17.3199, -7.0125) ccw
  arc A443 (23.4022, -0.7958) -> (23.5404, -0.4211) centre (4.2393, 6.4866) ccw
  arc A444 (22.9161, -0.8038) -> (23.4022, -0.7958) centre (23.034, 6.7826) ccw
  arc A445 (22.5226, -0.7856) -> (22.9161, -0.8038) centre (23.0153, 5.6031) ccw
  arc A446 (22.0661, -1.1027) -> (22.2112, -0.7523) centre (4.2393, 6.4866) ccw
  arc A447 (22.2112, -0.7523) -> (22.5226, -0.7856) centre (22.9275, 4.4707) ccw
  arc A448 (22.865, 0.1425) -> (22.6065, 0.3194) centre (19.7592, -4.1175) ccw
  arc A449 (23.1761, -0.0993) -> (22.865, 0.1425) centre (19.0905, -5.0356) ccw
  arc A450 (23.5404, -0.4211) -> (23.1761, -0.0993) centre (18.3387, -5.9446) ccw
  arc A451 (23.9145, 0.7301) -> (24.0229, 1.1146) centre (4.2393, 6.4866) ccw
  arc A452 (23.4306, 0.684) -> (23.9145, 0.7301) centre (22.9529, 8.2563) ccw
  arc A453 (23.0368, 0.6713) -> (23.4306, 0.684) centre (23.0268, 7.079) ccw
  arc A454 (22.6065, 0.3194) -> (22.7237, 0.6801) centre (4.2393, 6.4866) ccw
  arc A455 (22.7237, 0.6801) -> (23.0368, 0.6713) centre (23.0281, 5.9432) ccw
  arc A456 (23.3053, 1.6234) -> (23.0338, 1.7794) centre (20.5433, -2.8671) ccw
  arc A457 (23.6344, 1.4068) -> (23.3053, 1.6234) centre (19.9488, -3.8349) ccw
  arc A458 (24.0229, 1.1146) -> (23.6344, 1.4068) centre (19.2706, -4.8001) ccw
  arc A459 (24.3055, 2.2916) -> (24.3834, 2.6834) centre (4.2393, 6.4866) ccw
  arc A460 (23.8267, 2.2076) -> (24.3055, 2.2916) centre (22.7564, 9.7191) ccw
  arc A461 (23.4351, 2.164) -> (23.8267, 2.2076) centre (22.9224, 8.5512) ccw
  arc A462 (23.0338, 1.7794) -> (23.1223, 2.1482) centre (4.2393, 6.4866) ccw
  arc A463 (23.1223, 2.1482) -> (23.4351, 2.164) centre (23.0128, 7.419) ccw
  arc A464 (23.6281, 3.1343) -> (23.3452, 3.2686) centre (21.2269, -1.5591) ccw
  arc A465 (23.9732, 2.9442) -> (23.6281, 3.1343) centre (20.7102, -2.5705) ccw
  arc A466 (24.3834, 2.6834) -> (23.9732, 2.9442) centre (20.1098, -3.5859) ccw
  arc A467 (24.5728, 3.8789) -> (24.6197, 4.2756) centre (4.2393, 6.4866) ccw
  arc A468 (24.102, 3.7576) -> (24.5728, 3.8789) centre (22.4457, 11.1619) ccw
  arc A469 (23.7151, 3.6834) -> (24.102, 3.7576) centre (22.7028, 10.0107) ccw
  arc A470 (23.3452, 3.2686) -> (23.4045, 3.6431) centre (4.2393, 6.4866) ccw
  arc A471 (23.4045, 3.6431) -> (23.7151, 3.6834) centre (22.8818, 8.8891) ccw
  arc A472 (23.8314, 4.6658) -> (23.5388, 4.7775) centre (21.8058, -0.2015) ccw
  arc A473 (24.1903, 4.5034) -> (23.8314, 4.6658) centre (21.37, -1.2503) ccw
  arc A474 (24.6197, 4.2756) -> (24.1903, 4.5034) centre (20.8512, -2.3097) ccw
  arc A475 (24.7147, 5.4823) -> (24.7304, 5.8814) centre (4.2393, 6.4866) ccw
  arc A476 (24.2549, 5.3244) -> (24.7147, 5.4823) centre (22.0227, 12.576) ccw
  arc A477 (23.875, 5.2201) -> (24.2549, 5.3244) centre (22.3694, 11.4485) ccw
  arc A478 (23.5388, 4.7775) -> (23.5685, 5.1556) centre (4.2393, 6.4866) ccw
  arc A479 (23.5685, 5.1556) -> (23.875, 5.2201) centre (22.6358, 10.3443) ccw
  arc A480 (23.9138, 6.2086) -> (23.6134, 6.297) centre (22.2764, 1.1974) ccw
  arc A481 (24.2844, 6.0748) -> (23.9138, 6.2086) centre (21.9242, 0.1176) ccw
  arc A482 (24.7304, 5.8814) -> (24.2844, 6.0748) centre (21.4901, -0.9792) ccw
  arc A483 (24.7304, 7.0918) -> (24.7147, 7.491) centre (4.2393, 6.4866) ccw
  arc A484 (24.2844, 6.8984) -> (24.7304, 7.0918) centre (21.4901, 13.9525) ccw
  arc A485 (23.9138, 6.7646) -> (24.2844, 6.8984) centre (21.9242, 12.8556) ccw
  arc A486 (23.6134, 6.297) -> (23.6134, 6.6762) centre (4.2393, 6.4866) ccw
  arc A487 (23.6134, 6.6762) -> (23.9138, 6.7646) centre (22.2764, 11.7758) ccw
  arc A488 (23.875, 7.7531) -> (23.5685, 7.8177) centre (22.6358, 2.6289) ccw
  arc A489 (24.2549, 7.6488) -> (23.875, 7.7531) centre (22.3694, 1.5248) ccw
  arc A490 (24.7147, 7.491) -> (24.2549, 7.6488) centre (22.0227, 0.3973) ccw
  arc A491 (24.6197, 8.6977) -> (24.5728, 9.0944) centre (4.2393, 6.4866) ccw
  arc A492 (24.1903, 8.4699) -> (24.6197, 8.6977) centre (20.8512, 15.2829) ccw
  arc A493 (23.8314, 8.3074) -> (24.1903, 8.4699) centre (21.37, 14.2235) ccw
  arc A494 (23.5685, 7.8177) -> (23.5388, 8.1957) centre (4.2393, 6.4866) ccw
  arc A495 (23.5388, 8.1957) -> (23.8314, 8.3074) centre (21.8058, 13.1747) ccw
  arc A496 (23.7151, 9.2898) -> (23.4045, 9.3301) centre (22.8818, 4.0842) ccw
  arc A497 (24.102, 9.2156) -> (23.7151, 9.2898) centre (22.7028, 2.9626) ccw
  arc A498 (24.5728, 9.0944) -> (24.102, 9.2156) centre (22.4457, 1.8113) ccw
  arc A499 (24.3834, 10.2899) -> (24.3055, 10.6817) centre (4.2393, 6.4866) ccw
  arc A500 (23.9732, 10.0291) -> (24.3834, 10.2899) centre (20.1098, 16.5592) ccw
  arc A501 (23.6281, 9.839) -> (23.9732, 10.0291) centre (20.7102, 15.5438) ccw
  arc A502 (23.4045, 9.3301) -> (23.3452, 9.7047) centre (4.2393, 6.4866) ccw
  arc A503 (23.3452, 9.7047) -> (23.6281, 9.839) centre (21.2269, 14.5323) ccw
  arc A504 (23.4351, 10.8092) -> (23.1223, 10.825) centre (23.0128, 5.5542) ccw
  arc A505 (23.8267, 10.7656) -> (23.4351, 10.8092) centre (22.9224, 4.422) ccw
  arc A506 (24.3055, 10.6817) -> (23.8267, 10.7656) centre (22.7564, 3.2542) ccw
  arc A507 (24.0229, 11.8587) -> (23.9145, 12.2431) centre (4.2393, 6.4866) ccw
  arc A508 (23.6344, 11.5665) -> (24.0229, 11.8587) centre (19.2706, 17.7733) ccw
  arc A509 (23.3053, 11.3499) -> (23.6344, 11.5665) centre (19.9488, 16.8081) ccw
  arc A510 (23.1223, 10.825) -> (23.0338, 11.1938) centre (4.2393, 6.4866) ccw
  arc A511 (23.0338, 11.1938) -> (23.3053, 11.3499) centre (20.5433, 15.8404) ccw
  arc A512 (23.0368, 12.302) -> (22.7237, 12.2932) centre (23.0281, 7.0301) ccw
  arc A513 (23.4306, 12.2893) -> (23.0368, 12.302) centre (23.0268, 5.8943) ccw
  arc A514 (23.9145, 12.2431) -> (23.4306, 12.2893) centre (22.9529, 4.717) ccw
  arc A515 (23.5404, 13.3943) -> (23.4022, 13.7691) centre (4.2393, 6.4866) ccw
  arc A516 (23.1761, 13.0725) -> (23.5404, 13.3943) centre (18.3387, 18.9179) ccw
  arc A517 (22.865, 12.8308) -> (23.1761, 13.0725) centre (19.0905, 18.0089) ccw
  arc A518 (22.7237, 12.2932) -> (22.6065, 12.6539) centre (4.2393, 6.4866) ccw
  arc A519 (22.6065, 12.6539) -> (22.865, 12.8308) centre (19.7592, 17.0907) ccw
  arc A520 (22.5226, 13.7589) -> (22.2112, 13.7256) centre (22.9275, 8.5025) ccw
  arc A521 (22.9161, 13.7771) -> (22.5226, 13.7589) centre (23.0153, 7.3701) ccw
  arc A522 (23.4022, 13.7691) -> (22.9161, 13.7771) centre (23.034, 6.1907) ccw
  arc A523 (22.939, 14.8874) -> (22.7717, 15.2501) centre (4.2393, 6.4866) ccw
  arc A524 (22.601, 14.538) -> (22.939, 14.8874) centre (17.3199, 19.9858) ccw
  arc A525 (22.3098, 14.2726) -> (22.601, 14.538) centre (18.1407, 19.1385) ccw
  arc A526 (22.2112, 13.7256) -> (22.0661, 14.076) centre (4.2393, 6.4866) ccw
  arc A527 (22.0661, 14.076) -> (22.3098, 14.2726) centre (18.8793, 18.2757) ccw
  arc A528 (21.8956, 15.171) -> (21.5878, 15.1133) centre (22.7117, 9.9626) ccw
  arc A529 (22.2866, 15.22) -> (21.8956, 15.171) centre (22.8881, 8.8406) ccw
  arc A530 (22.7717, 15.2501) -> (22.2866, 15.22) centre (22.9993, 7.6662) ccw
  arc A531 (22.2222, 16.3286) -> (22.027, 16.6771) centre (4.2393, 6.4866) ccw
  arc A532 (21.9127, 15.9538) -> (22.2222, 16.3286) centre (16.2205, 20.9705) ccw
  arc A533 (21.6432, 15.6664) -> (21.9127, 15.9538) centre (17.1052, 20.1902) ccw
  arc A534 (21.5878, 15.1133) -> (21.4156, 15.4512) centre (4.2393, 6.4866) ccw
  arc A535 (21.4156, 15.4512) -> (21.6432, 15.6664) centre (17.9092, 19.388) ccw
  arc A536 (21.1598, 16.5295) -> (20.8575, 16.4479) centre (22.3821, 11.4012) ccw
  arc A537 (21.5457, 16.609) -> (21.1598, 16.5295) centre (22.646, 10.2965) ccw
  arc A538 (22.027, 16.6771) -> (21.5457, 16.609) centre (22.8489, 9.1345) ccw
  arc A539 (21.3946, 17.7092) -> (21.1727, 18.0413) centre (4.2393, 6.4866) ccw
  arc A540 (21.1154, 17.3113) -> (21.3946, 17.7092) centre (15.0472, 21.8658) ccw
  arc A541 (20.8693, 17.0036) -> (21.1154, 17.3113) centre (15.9904, 21.1574) ccw
  arc A542 (20.8575, 16.4479) -> (20.6593, 16.7712) centre (4.2393, 6.4866) ccw
  arc A543 (20.6593, 16.7712) -> (20.8693, 17.0036) centre (16.8549, 20.4208) ccw
  arc A544 (20.3197, 17.8261) -> (20.0247, 17.721) centre (21.9406, 12.8095) ccw
  arc A545 (20.6982, 17.9357) -> (20.3197, 17.8261) centre (22.2903, 11.7289) ccw
  arc A546 (21.1727, 18.0413) -> (20.6982, 17.9357) centre (22.5838, 10.5864) ccw
  arc A547 (20.4612, 19.0206) -> (20.2139, 19.3343) centre (4.2393, 6.4866) ccw
  arc A548 (20.2141, 18.602) -> (20.4612, 19.0206) centre (13.8072, 22.6664) ccw
  arc A549 (19.9929, 18.2759) -> (20.2141, 18.602) centre (14.8031, 22.0342) ccw
  arc A550 (20.0247, 17.721) -> (19.8018, 18.0278) centre (4.2393, 6.4866) ccw
  arc A551 (19.8018, 18.0278) -> (19.9929, 18.2759) centre (15.7227, 21.3676) ccw
  arc A552 (19.3805, 19.0528) -> (19.0946, 18.9249) centre (21.3899, 14.1788) ccw
  arc A553 (19.7492, 19.1917) -> (19.3805, 19.0528) centre (21.8234, 13.129) ccw
  arc A554 (20.2139, 19.3343) -> (19.7492, 19.1917) centre (22.2056, 12.0131) ccw
  arc A555 (19.4278, 20.2547) -> (19.1566, 20.548) centre (4.2393, 6.4866) ccw
  arc A556 (19.2143, 19.818) -> (19.4278, 20.2547) centre (12.5083, 23.3672) ccw
  arc A557 (19.0194, 19.4756) -> (19.2143, 19.818) centre (13.5507, 22.8151) ccw
  arc A558 (19.0946, 18.9249) -> (18.8483, 19.2133) centre (4.2393, 6.4866) ccw
  arc A559 (18.8483, 19.2133) -> (19.0194, 19.4756) centre (14.5198, 22.2227) ccw
  arc A560 (18.3479, 20.202) -> (18.0729, 20.0521) centre (20.7335, 15.5007) ccw
  arc A561 (18.7045, 20.3695) -> (18.3479, 20.202) centre (21.248, 14.4882) ccw
  arc A562 (19.1566, 20.548) -> (18.7045, 20.3695) centre (21.7166, 13.4056) ccw
  arc A563 (18.3007, 21.4039) -> (18.0074, 21.6751) centre (4.2393, 6.4866) ccw
  arc A564 (18.1221, 20.9518) -> (18.3007, 21.4039) centre (11.1583, 23.964) ccw
  arc A565 (17.9547, 20.5952) -> (18.1221, 20.9518) centre (12.2409, 23.4953) ccw
  arc A566 (18.0729, 20.0521) -> (17.8048, 20.3202) centre (4.2393, 6.4866) ccw
  arc A567 (17.8048, 20.3202) -> (17.9547, 20.5952) centre (13.2534, 22.9808) ccw
  arc A568 (17.2283, 21.2667) -> (16.966, 21.0956) centre (19.9754, 16.7671) ccw
  arc A569 (17.5707, 21.4616) -> (17.2283, 21.2667) centre (20.5678, 15.798) ccw
  arc A570 (18.0074, 21.6751) -> (17.5707, 21.4616) centre (21.1199, 14.7556) ccw
  arc A571 (17.087, 22.4612) -> (16.7733, 22.7085) centre (4.2393, 6.4866) ccw
  arc A572 (16.9444, 21.9965) -> (17.087, 22.4612) centre (9.7657, 24.4529) ccw
  arc A573 (16.8055, 21.6278) -> (16.9444, 21.9965) centre (10.8817, 24.0707) ccw
  arc A574 (16.966, 21.0956) -> (16.6776, 21.3419) centre (4.2393, 6.4866) ccw
  arc A575 (16.6776, 21.3419) -> (16.8055, 21.6278) centre (11.9315, 23.6372) ccw
  arc A576 (16.0286, 22.2402) -> (15.7805, 22.0491) centre (19.1203, 17.97) ccw
  arc A577 (16.3547, 22.4614) -> (16.0286, 22.2402) centre (19.7869, 17.0504) ccw
  arc A578 (16.7733, 22.7085) -> (16.3547, 22.4614) centre (20.4191, 16.0545) ccw
  arc A579 (15.794, 23.42) -> (15.4619, 23.6419) centre (4.2393, 6.4866) ccw
  arc A580 (15.6884, 22.9455) -> (15.794, 23.42) centre (8.3391, 24.8311) ccw
  arc A581 (15.5788, 22.567) -> (15.6884, 22.9455) centre (9.4816, 24.5376) ccw
  arc A582 (15.7805, 22.0491) -> (15.4737, 22.272) centre (4.2393, 6.4866) ccw
  arc A583 (15.4737, 22.272) -> (15.5788, 22.567) centre (10.5622, 24.1879) ccw
  arc A584 (14.7563, 23.1166) -> (14.5239, 22.9067) centre (18.1735, 19.1022) ccw
  arc A585 (15.064, 23.3627) -> (14.7563, 23.1166) centre (18.9101, 18.2377) ccw
  arc A586 (15.4619, 23.6419) -> (15.064, 23.3627) centre (19.6185, 17.2945) ccw
  arc A587 (14.4298, 24.2743) -> (14.0813, 24.4695) centre (4.2393, 6.4866) ccw
  arc A588 (14.3617, 23.793) -> (14.4298, 24.2743) centre (6.8872, 25.0963) ccw
  arc A589 (14.2822, 23.4072) -> (14.3617, 23.793) centre (8.0492, 24.8933) ccw
  arc A590 (14.5239, 22.9067) -> (14.2006, 23.1048) centre (4.2393, 6.4866) ccw
  arc A591 (14.2006, 23.1048) -> (14.2822, 23.4072) centre (9.1539, 24.6294) ccw
  arc A592 (13.4191, 23.8905) -> (13.2039, 23.663) centre (17.1407, 20.1566) ccw
  arc A593 (13.7065, 24.16) -> (13.4191, 23.8905) centre (17.9429, 19.3525) ccw
  arc A594 (14.0813, 24.4695) -> (13.7065, 24.16) centre (18.7231, 18.4678) ccw
  arc A595 (13.0028, 25.0191) -> (12.64, 25.1863) centre (4.2393, 6.4866) ccw
  arc A596 (12.9727, 24.5339) -> (13.0028, 25.0191) centre (5.4189, 25.2466) ccw
  arc A597 (12.9236, 24.143) -> (12.9727, 24.5339) centre (6.5933, 25.1355) ccw
  arc A598 (13.2039, 23.663) -> (12.866, 23.8351) centre (4.2393, 6.4866) ccw
  arc A599 (12.866, 23.8351) -> (12.9236, 24.143) centre (7.7153, 24.9591) ccw
  arc A600 (12.0253, 24.5571) -> (11.8286, 24.3134) centre (16.0284, 21.1266) ccw
  arc A601 (12.2907, 24.8483) -> (12.0253, 24.5571) centre (16.8912, 20.388) ccw
  arc A602 (12.64, 25.1863) -> (12.2907, 24.8483) centre (17.7385, 19.5672) ccw
  arc A603 (11.5218, 25.6495) -> (11.147, 25.7878) centre (4.2393, 6.4866) ccw
  arc A604 (11.5298, 25.1635) -> (11.5218, 25.6495) centre (3.9434, 25.2814) ccw
  arc A605 (11.5116, 24.7699) -> (11.5298, 25.1635) centre (5.1228, 25.2627) ccw
  arc A606 (11.8286, 24.3134) -> (11.4783, 24.4585) centre (4.2393, 6.4866) ccw
  arc A607 (11.4783, 24.4585) -> (11.5116, 24.7699) centre (6.2552, 25.1748) ccw